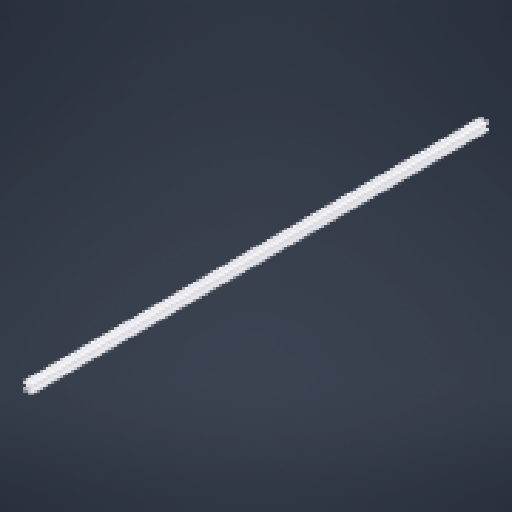
# Autodesk Inventor part: PERFIL 2020 V-SLOT
Saved by Autodesk Inventor 2026.2 (Build 302298000, 298)
## iProperties
Created: 1705-05-12
Part Number: PERFIL 2020 V-SLOT
Material: 6063-T5
Document SubType Name: Modeling
Designer: Ian
Density: 2.7 g/cm^3
Appearance: satin finish aluminum
Part Number: PF20-11 - PERFIL 2020 V-SLOT
Sending System: SOLIDWORKS 2019
Componente: PF20-11 - PERFIL 2020 V-SLOT
Last Saved Date: 2022-03-25
last saved by: pd
Author: Ian
Autodesk Inventor part; units mm, degrees
ref_plane "YZ Plane" through (0, 0, 0) normal (1, 0, 0) x (0, 1, 0)
ref_plane "Plano1" through (0, 0, -500) normal (0, 0, 1) x (1, 0, 0)
ref_plane "Plano de trabalho2" through (-9, -10, 500) normal (0, 0, 1) x (1, 0, 0)
sketch "Esboço1" plane through (-9, -10, 500) normal (0, 0, 1) x (1, 0, 0)
  arc A0 (-1, 1) -> (0, 0) centre (0, 1) ccw projected
  line L0 (0, 0) -> (4.2, 0) projected
  line L1 (4.2, 0) -> (6, 1.8) projected
  line L2 (6, 1.8) -> (3.5, 1.8) projected
  line L3 (3.5, 1.8) -> (3.5, 3.4393) projected
  line L4 (3.5, 3.4393) -> (6.0607, 6) projected
  line L5 (6.0607, 6) -> (8.7, 6) projected
  line L6 (8.7, 6) -> (9, 6.3) projected
  line L7 (9, 6.3) -> (9.3, 6) projected
  line L8 (9.3, 6) -> (11.9393, 6) projected
  line L9 (11.9393, 6) -> (14.5, 3.4393) projected
  line L10 (14.5, 3.4393) -> (14.5, 1.8) projected
  line L11 (14.5, 1.8) -> (12, 1.8) projected
  line L12 (12, 1.8) -> (13.8, 0) projected
  line L13 (13.8, 0) -> (18, 0) projected
  arc A1 (18, 0) -> (19, 1) centre (18, 1) ccw projected
  line L14 (19, 1) -> (19, 5.2) projected
  line L15 (19, 5.2) -> (17.2, 7) projected
  line L16 (17.2, 7) -> (17.2, 4.5) projected
  line L17 (17.2, 4.5) -> (15.5607, 4.5) projected
  line L18 (15.5607, 4.5) -> (13, 7.0607) projected
  line L19 (13, 7.0607) -> (13, 9.7) projected
  line L20 (13, 9.7) -> (12.7, 10) projected
  line L21 (12.7, 10) -> (13, 10.3) projected
  line L22 (13, 10.3) -> (13, 12.9393) projected
  line L23 (13, 12.9393) -> (15.5607, 15.5) projected
  line L24 (15.5607, 15.5) -> (17.2, 15.5) projected
  line L25 (17.2, 15.5) -> (17.2, 13) projected
  line L26 (17.2, 13) -> (19, 14.8) projected
  line L27 (19, 14.8) -> (19, 19) projected
  arc A2 (19, 19) -> (18, 20) centre (18, 19) ccw projected
  line L28 (18, 20) -> (13.8, 20) projected
  line L29 (13.8, 20) -> (12, 18.2) projected
  line L30 (12, 18.2) -> (14.5, 18.2) projected
  line L31 (14.5, 18.2) -> (14.5, 16.5607) projected
  line L32 (14.5, 16.5607) -> (11.9393, 14) projected
  line L33 (11.9393, 14) -> (9.3, 14) projected
  line L34 (9.3, 14) -> (9, 13.7) projected
  line L35 (9, 13.7) -> (8.7, 14) projected
  line L36 (8.7, 14) -> (6.0607, 14) projected
  line L37 (6.0607, 14) -> (3.5, 16.5607) projected
  line L38 (3.5, 16.5607) -> (3.5, 18.2) projected
  line L39 (3.5, 18.2) -> (6, 18.2) projected
  line L40 (6, 18.2) -> (4.2, 20) projected
  line L41 (4.2, 20) -> (0, 20) projected
  arc A3 (0, 20) -> (-1, 19) centre (0, 19) ccw projected
  line L42 (-1, 19) -> (-1, 14.8) projected
  line L43 (-1, 14.8) -> (0.8, 13) projected
  line L44 (0.8, 13) -> (0.8, 15.5) projected
  line L45 (0.8, 15.5) -> (2.4393, 15.5) projected
  line L46 (2.4393, 15.5) -> (5, 12.9393) projected
  line L47 (5, 12.9393) -> (5, 10.3) projected
  line L48 (5, 10.3) -> (5.3, 10) projected
  line L49 (5.3, 10) -> (5, 9.7) projected
  line L50 (5, 9.7) -> (5, 7.0607) projected
  line L51 (5, 7.0607) -> (2.4393, 4.5) projected
  line L52 (2.4393, 4.5) -> (0.8, 4.5) projected
  line L53 (0.8, 4.5) -> (0.8, 7) projected
  line L54 (0.8, 7) -> (-1, 5.2) projected
  line L55 (-1, 5.2) -> (-1, 1) projected
  circle A4 centre (9, 10) radius 2.3 projected
extrude "Extrusão1" add sketch "Esboço1" along normal blind 1080
